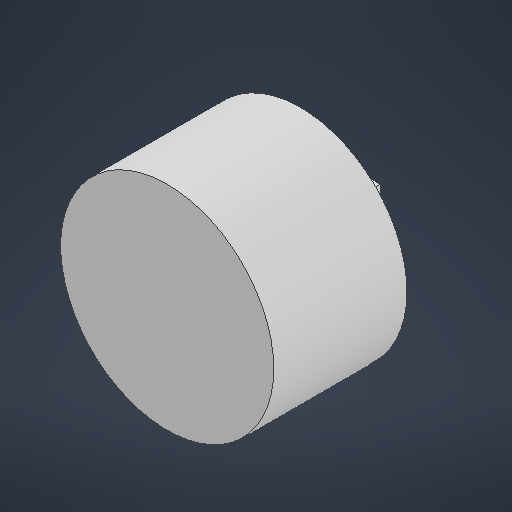
# Autodesk Inventor part: Shaft-EndCap
Saved by Autodesk Inventor 2026.1 (Build 301233000, 233)
## iProperties
Created: 2025-11-04
Part Number: Shaft-EndCap
Material: Generic
Document SubType Name: Modeling
Designer: uu-112
Density: 1 g/cm^3
Appearance: Default
Author: uu-112
Autodesk Inventor part; units mm, degrees
ref_plane "YZ Plane" through (0, 0, 0) normal (1, 0, 0) x (0, 1, 0)
ref_plane "XZ Plane" through (0, 0, 0) normal (0, 1, 0) x (-1, 0, 0)
ref_plane "XY Plane" through (0, 0, 0) normal (0, 0, 1) x (1, 0, 0)
sketch "Sketch1" plane through (0, 0, 0) normal (0, 0, 1) x (1, 0, 0)
  line L0 (2.54, -2.54) -> (-2.54, -2.54)
  line L1 (-2.54, -2.54) -> (-2.54, 2.54)
  line L2 (-2.54, 2.54) -> (2.54, 2.54)
  line L3 (2.54, 2.54) -> (2.54, -2.54)
  line L4 (2.54, -2.54) -> (-2.54, 2.54) construction
  line L5 (-2.54, -2.54) -> (2.54, 2.54) construction
  point P0 (0, 0)
  dimension "d0" = 5.08
  dimension "d1" = 5.08
  constraints: 12 end point, 2 midpoint, 2 parallel, 1 horizontal, 1 perpendicular
  measures "d0" distance of L1.end L2.end
  measures "d1" distance of L0.end L1.end
extrude "Extrusion1" add sketch "Sketch1" along normal mid plane 3.175
sketch "Sketch2" plane through (0, 0, 1.5875) normal (0, 0, 1) x (1, 0, 0)
  circle A0 centre (0, 0) radius 7.62
  dimension "d4" = 15.24
  constraints: 1 centre point, 1 coincident
  measures "d4" diameter of A0
extrude "Extrusion2" add sketch "Sketch2" along normal blind 9.525
body "Solid1"
